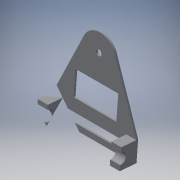
# Autodesk Inventor part: soporte worm
Saved by Autodesk Inventor 2016 (Build 200138000, 138)
## iProperties
Created: 2016-07-30
Part Number: soporte worm
Material: Generic
Document SubType Name: Modeling
Designer: Admin
Density: 1 g/cm^3
Appearance: Default
Author: Admin
Autodesk Inventor part; units mm, degrees
ref_plane "YZ Plane" through (0, 0, 0) normal (1, 0, 0) x (0, 1, 0)
ref_plane "XZ Plane" through (0, 0, 0) normal (0, 1, 0) x (-1, 0, 0)
ref_plane "XY Plane" through (0, 0, 0) normal (0, 0, 1) x (1, 0, 0)
ref_plane "Work Plane1" through (165.2318, -51.2393, 94.4671) normal (0, 0.9967757, -0.0802378) x (1, 0, 0)
sketch "Sketch1" plane through (165.2318, -51.2393, 94.4671) normal (0, 0.9967757, -0.0802378) x (1, 0, 0)
  circle A0 centre (-3, -0.1506) radius 18.8079
  line L0 (-49, 58) -> (43, 58)
  line L1 (43, 58) -> (43, 80)
  line L2 (43, 80) -> (-49, 80)
  line L3 (-49, 80) -> (-49, 58)
  line L4 (-19.1864, -9.7285) -> (-49, 58)
  line L5 (13.1864, -9.7285) -> (43, 58)
  line L6 (-26.5, 26) -> (20.5, 26)
  line L7 (20.5, 26) -> (20.5, 52)
  line L8 (20.5, 52) -> (-26.5, 52)
  line L9 (-26.5, 52) -> (-26.5, 26)
  line L10 (-44, 65) -> (39, 65)
  line L11 (39, 65) -> (39, 74)
  line L12 (39, 74) -> (-44, 74)
  line L13 (-44, 74) -> (-44, 65)
  circle A1 centre (-3, -0.1506) radius 3
  point P0 (-165.2318, 90.0511)
  dimension "d2" = 6
  dimension "d13" = 74
  dimension "d14" = 74
  dimension "d15" = 22.5
  dimension "d16" = 22.5
  dimension "d17" = 23.5
  dimension "d18" = 23.5
  constraints: 28 end point, 6 parallel, 3 horizontal, 3 perpendicular, 2 centre point, 2 point on circle, 1 coincident
  measures "d2" diameter of A1
  measures "d13" distance of L4.start L0.start
  measures "d14" distance of L5.start L0.end
  measures "d15" distance between parallel lines of L1 L7
  measures "d16" distance between parallel lines of L3 L9
  measures "d17" distance from line of L7 A1.centre
  measures "d18" distance from line of L9 A0.centre
extrude "Extrusion2" add sketch "Sketch1" along normal blind 2 contours L4 A0 L5 | L4 L0 L5 A0 | L3 L2 L1 L0
sketch "Sketch2" plane through (165.2318, -51.2393, 94.4671) normal (0, -0.9967757, 0.0802378) x (1, 0, 0)
  line L0 (43, -80) -> (-49, -80) projected
  line L1 (-49, -58) -> (-38, -58)
  line L2 (-38, -58) -> (-38, -80)
  line L3 (-38, -80) -> (-49, -80)
  line L4 (-49, -80) -> (-49, -58)
  line L5 (43, -58) -> (43, -80) projected
  line L6 (43, -58) -> (32, -58)
  line L7 (32, -58) -> (32, -80)
  line L8 (32, -80) -> (43, -80)
  line L9 (43, -80) -> (43, -58)
  point P0 (-165.2318, -90.0511)
  dimension "d19" = 11
  dimension "d20" = 11
  constraints: 16 end point, 4 parallel, 2 horizontal, 2 perpendicular, 2 point on line
  measures "d19" distance of L1.start L1.end
  measures "d20" distance of L5.start L6.end
extrude "Extrusion3" add sketch "Sketch2" along normal blind 16.5
sketch "Sketch4" plane through (116.2318, -55.6648, 14.5645) normal (-1, 0, 0) x (0, 0.0802378, 0.9967757)
  line L0 (22, -18.5) -> (0, -18.5) projected
  circle A0 centre (11.5, -18.5) radius 6
  point P0 (-10.0511, 56.6539)
  dimension "d10" = 12
  constraints: 1 centre point, 1 point on line
  measures "d10" diameter of A0
extrude "Extrusion5" cut sketch "Sketch4" against normal through all
body "Solid2"
